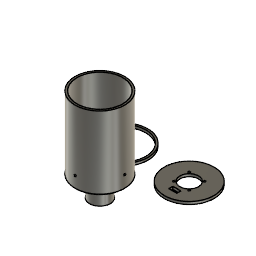
enclosure (Autodesk Fusion 360 design; units mm, degrees)
part number: 2025-12-08-12-09-59-387
part number: 2025-12-08-12-10-12-289
Autodesk Fusion 360 part; units mm, degrees
note: some values were not read from the file. Set by a fixed rule: which face or edge a step refers to.
sketch "Sketch1" plane through (0, 0, 0) normal (0, 0, 1) x (1, 0, 0) in component "Component"
  circle A0 centre (0, 0) radius 37.5
  circle A1 centre (0, 0) radius 13
  dimension "d1" = 75
  dimension "d2" = 26
  constraint coincident A0.centre A1.centre
  measures "d1" diameter of A0
  measures "d2" diameter of A1
extrude "Extrude1" add sketch "Sketch1" against normal blind 10 makes body 1 in component "Component"
sketch "Sketch2" plane through (0, 0, 0) normal (0, 0, 1) x (1, 0, 0) in component "Component"
  circle A0 centre (0, 0) radius 13
  circle A1 centre (0, 0) radius 15.8
  circle A2 centre (0, 0) radius 13
  dimension "d11" = 31.6
  dimension "d12" = 26
  constraint concentric A0 A1
  constraint concentric A0 A2
  measures "d11" diameter of A1
  measures "d12" diameter of A2
extrude "Extrude2" add sketch "Sketch2" along normal blind 30 bodies 1 in component "Component"
fillet "Fillet1" radius 2 1 edges at (-14.7308, 5.7135, 0) on bodies 1 in component "Component"
sketch "Sketch3" plane through (0, 0, -10) normal (0, 0, -1) x (1, 0, 0) in component "Component"
  circle A0 centre (0, 0) radius 13
  circle A1 centre (0, 0) radius 37.5
  circle A2 centre (0, 0) radius 37.5
  circle A3 centre (0, 0) radius 34.5
  dimension "d17" = -3
extrude "Extrude3" add sketch "Sketch3" along normal blind 50 contours A1 A2 bodies 1 in component "Component"
sketch "Sketch4" plane through (0, 0, 0) normal (0, 0, 1) x (1, 0, 0) in component "Component"
extrude "Extrude4" add 1 faces at (36.3604, 1.863, -60) along direction (0, 0, -1) blind 50 on bodies 1 bodies 1 in component "Component"
sketch "Sketch5" plane through (0, 0, 0) normal (0, 1, 0) x (1, 0, 0) in component "Component"
hole "Hole1" at (37.5, 0, -18.9437) direction (-1, 0, 0) diameter 3 depth 50 tip angle 118 bodies 1 in component "Component"
hole "Hole2" at (0, 37.5, -17.7105) direction (0, -1, 0) diameter 3 depth 50 tip angle 118 bodies 1 in component "Component"
hole "Hole3" at (0, -37.5, -18.8569) direction (0, 1, 0) diameter 3 depth 50 tip angle 118 bodies 1 in component "Component"
sketch "Sketch6" plane through (0, 0, -110) normal (0, 0, -1) x (1, 0, 0) in component "Component"
  circle A0 centre (0, 0) radius 34.5
  circle A1 centre (0, 0) radius 37.5
  circle A2 centre (0, 0) radius 34.5
  circle A3 centre (0, 0) radius 37.5
extrude "Extrude5" add sketch "Sketch6" against normal blind 4 separate body makes body 2 in component "Component"
fillet "Fillet2" radius 0.2 1 edges at (-34.9623, 13.5606, -110) on bodies 2 in component "Component"
extrude "Extrude6" add sketch "Sketch6" against normal blind 4 separate body contours A0 A2 | A1 A3 makes body 3 in component "Component"
sketch "Sketch7" plane through (0, 0, -110) normal (0, 0, -1) x (1, 0, 0) in component "Component"
  circle A0 centre (0, 0) radius 14
  line L0 (-14, 14) -> (14, 14)
  line L1 (14, 14) -> (14, -14)
  line L2 (14, -14) -> (-14, -14)
  line L3 (-14, -14) -> (-14, 14)
  line L4 (-14, 14) -> (14, -14) construction
  line L5 (14, 14) -> (-14, -14) construction
  circle A1 centre (-11.5917, 11.5917) radius 1.5
  circle A2 centre (11.5887, 11.5887) radius 1.5
  circle A3 centre (-12, -12) radius 1.5
  circle A4 centre (11.6655, -11.6655) radius 1.5
  dimension "d37" = 28
  dimension "d38" = 28
  dimension "d39" = 28
  dimension "d40" = 3
  dimension "d41" = 3
  dimension "d42" = 3
  dimension "d43" = 3
  constraint coincident A0.centre origin
  constraint horizontal L0
  constraint perpendicular L0 L1
  constraint parallel L0 L2
  constraint parallel L1 L3
  constraint coincident L4 A0.centre
  constraint coincident L5 A0.centre
  constraint coincident L4 A1.centre
  constraint coincident L5 A2.centre
  constraint coincident L5 A3.centre
  constraint coincident L4 A4.centre
  measures "d37" diameter of A0
  measures "d38" distance of L1.end L2.end
  measures "d39" distance of L0.end L1.end
  measures "d40" diameter of A1
  measures "d41" diameter of A2
  measures "d42" diameter of A3
  measures "d43" diameter of A4
extrude "Extrude7" cut sketch "Sketch7" against normal blind 4 contours A1 | A2 | A3 | A4 bodies 3 in component "Component"
extrude "Extrude8" cut sketch "Sketch7" against normal blind 4 contours A0 bodies 3 in component "Component"
sketch "Sketch8" plane through (0, 0, -110) normal (0, 0, -1) x (1, 0, 0) in component "Component"
  circle A0 centre (0, 0) radius 14
  circle A1 centre (-11.5917, 11.5917) radius 1.5
  circle A2 centre (11.6655, -11.6655) radius 1.5
  circle A3 centre (11.5887, 11.5887) radius 1.5
  circle A4 centre (-12, -12) radius 1.5
  circle A5 centre (0, 0) radius 37.5
  line L0 (-5.843, 25) -> (6.157, 25)
  line L1 (6.157, 25) -> (6.157, 19)
  line L2 (6.157, 19) -> (-5.843, 19)
  line L3 (-5.843, 19) -> (-5.843, 25)
  dimension "d48" = 12
  dimension "d49" = 6
  constraint horizontal L0
  constraint vertical L1
  constraint horizontal L2
  constraint vertical L3
  measures "d48" distance of L0.start L0.end
  measures "d49" distance of L0.start L2.end
extrude "Extrude9" cut sketch "Sketch8" against normal blind 5 contours L0 L1 L2 L3 bodies 3 in component "Component"
fillet "Fillet3" radius 1 1 edges at (-34.9623, -13.5606, 0) on bodies 1 in component "Component"
move_body "Move1" bodies 3 2 to x (1, 0, 0) y (0, 1, 0) z (0, 0, 1) at (0, 90, 120) in component "Component"
move_body "Move2" bodies 3 2 to x (1, 0, 0) y (0, 1, 0) z (0, 0, 1) at (0, 0, -15) in component "Component"
move_body "Move3" bodies 3 to x (1, 0, 0) y (0, 1, 0) z (0, 0, 1) at (90, 0, 0) in component "Component"
move_body "Move4" bodies 2 to x (1, 0, 0) y (0, 1, 0) z (0, 0, 1) at (-60, 0, 0) in component "Component"
move_body "Move5" bodies 3 to x (1, 0, 0) y (0, 1, 0) z (0, 0, 1) at (-50, 0, 0) in component "Component"
move_body "Move6" bodies 1 to x (-1, 0, 0) y (0, 1, 0) z (0, 0, -1) at (-75, 0, -220) in component "Component"
move_body "Move7" bodies 1 to x (1, 0, 0) y (0, 1, 0) z (0, 0, 1) at (0, 0, 100) in component "Component"
move_body "Move8" bodies 1 to x (1, 0, 0) y (0, 1, 0) z (0, 0, 1) at (0, 0, 10) in component "Component"
move_body "Move9" bodies 1 to x (1, 0, 0) y (0, 1, 0) z (0, 0, 1) at (60, 0, 0) in component "Component"
move_face "OffsetFaces1" offset 2.1 2 faces at (-27.9838, -0.648, -103.3333) (-27.9354, -1.2944, -130) on bodies 1 in component "Component"
move_face "OffsetFaces2" offset -2 2 faces at (-25.8865, -0.5433, -103.3333) (-25.8458, -1.0853, -130) on bodies 1 in component "Component"
move_face "OffsetFaces3" offset -1.5 2 faces at (-27.884, -0.643, -103.3333) (-27.8359, -1.2844, -130) on bodies 1 in component "Component"
move_face "OffsetFaces4" offset 0.7 2 faces at (-29.3821, -0.7178, -103.3333) (-29.3284, -1.4338, -130) on bodies 1 in component "Component"
move_face "OffsetFaces5" offset -0.7 2 faces at (-28.683, -0.6829, -103.3333) (-28.683, -0.6829, -120) on bodies 1 in component "Component"
move_face "OffsetFaces6" offset 0.7 2 faces at (-29.3821, -0.7178, -103.3333) (-29.3284, -1.4338, -130) on bodies 1 in component "Component"
move_face "OffsetFaces7" offset 0.7 2 faces at (-28.683, -0.6829, -103.3333) (-28.683, -0.6829, -120) on bodies 1 in component "Component"
move_face "OffsetFaces8" offset -1.4 2 faces at (-27.9838, -0.648, -103.3333) (-27.9354, -1.2944, -130) on bodies 1 in component "Component"
move_face "OffsetFaces9" offset 0.2 2 faces at (-29.3284, -1.4338, -106.6667) (-29.3821, -0.7178, -120) on bodies 1 in component "Component"
move_face "OffsetFaces10" offset 0.2 2 faces at (-29.1823, -0.7078, -103.3333) (-29.1294, -1.4139, -130) on bodies 1 in component "Component"
move_body "Move10" bodies 1 to x (1, 0, 0) y (0, -1, 0) z (0, 0, -1) at (0, -75.0028, -180) in component "Component"
move_body "Move11" bodies 1 to x (1, 0, 0) y (0, 1, 0) z (0, 0, 1) at (0, 0, 40) in component "Component"
move_body "Move12" bodies 1 to x (1, 0, 0) y (0, 1, 0) z (0, 0, 1) at (0, 80, 0) in component "Component"
move_body "Move13" bodies 2 to x (1, 0, 0) y (0, 1, 0) z (0, 0, 1) at (0, 0, 5) in component "Component"
move_body "Move14" bodies 3 to x (1, 0, 0) y (0, 1, 0) z (0, 0, 1) at (0, 0, 5) in component "Component"
move_body "Move15" bodies 1 to x (-1, 0, 0) y (0, 1, 0) z (0, 0, -1) at (-105.0028, 0, 15) in component "Component"
move_body "Move16" bodies 1 to x (1, 0, 0) y (0, 1, 0) z (0, 0, 1) at (0, 0, -15) in component "Component"
move_body "Move17" bodies 1 to x (1, 0, 0) y (0, 1, 0) z (0, 0, 1) at (80, 0, 0) in component "Component"
component "Component" placed x (1, 0, 0) y (0, 1, 0) z (0, 0, 1) at (0, 0, 0)
